test stack flex (Autodesk Fusion 360 design; units mm, degrees)
Autodesk Fusion 360 part; units mm, degrees
sketch "Sketch2" plane through (0, 0, 0) normal (0, 0, 1) x (1, 0, 0) in component "xy"
  line L0 (-95, 0) -> (-95, -95)
  line L1 (-95, -95) -> (0, -95)
  line L2 (0, -20) -> (0, 0)
  line L3 (-38, -95) -> (-38, -47)
  line L4 (-78, -95) -> (-78, -47)
  line L5 (0, 0) -> (-20, 0)
  line L6 (-20, 0) -> (-20, -20)
  line L7 (-20, -20) -> (0, -20)
  line L8 (0, -20) -> (0, 0)
  line L9 (-20, -20) -> (-68, -20)
  line L10 (-110, 0) -> (-110, -110)
  line L11 (-110, -110) -> (0, -110)
  line L12 (-68, -24) -> (-38, -43)
  line L13 (-38, -43) -> (-38, -47)
  line L14 (-38, -47) -> (-78, -47)
  line L15 (0, -95) -> (0, -110)
  line L16 (-95, 0) -> (-110, 0)
  line L17 (-95, 0) -> (-110, 0) construction
  line L18 (0, -110) -> (0, -95) construction
  line L19 (0, -20) -> (0, 0) construction
  line L20 (0, 0) -> (-110, 0) construction
  line L21 (-110, 0) -> (-110, -110) construction
  line L22 (-110, -110) -> (0, -110) construction
  line L23 (0, -110) -> (0, 0) construction
  line L24 (-58, -47) -> (-58, -95) construction
  line L25 (-58.625, -71) -> (-57.375, -71) construction
  line L26 (-58.625, -47) -> (-58.625, -95)
  line L27 (-57.375, -95) -> (-57.375, -47)
  line L28 (-39.25, -95) -> (-39.25, -47)
  line L29 (-76.75, -95) -> (-76.75, -47)
  line L30 (-20, -18.75) -> (-68, -18.75)
  line L31 (0, 0) -> (-20, 0)
  line L32 (-190, 0) -> (-210, 0) construction
  line L33 (-20, 0.625) -> (-68, 0.625)
  line L34 (-20, -0.625) -> (-68, -0.625)
  line L35 (-44, -0.625) -> (-44, 0.625) construction
  line L36 (-20, 0.625) -> (-20, 0)
  line L37 (-20, 18.75) -> (-68, 18.75)
  line L38 (-20, 20) -> (-68, 20)
  line L39 (-78, -47) -> (-78, 20)
  line L40 (-78, 20) -> (-68, 20)
  line L41 (-68, 20) -> (-68, -24)
  line L42 (-20, 18.75) -> (-20, 20)
  line L43 (-20, 20) -> (-20, -18.75)
  line L44 (-20, -20) -> (20, -20)
  line L45 (20, -20) -> (20, 20)
  line L46 (20, 20) -> (-20, 20)
  line L47 (-20, 20) -> (-20, -20)
  line L48 (-20, -20) -> (20, 20) construction
  line L49 (20, -20) -> (-20, 20) construction
  point P0 (-44, 0)
  dimension "d47" = 40
  dimension "d48" = 17
  dimension "d52" = 15
  dimension "d56" = 4
  dimension "d57" = 110
  dimension "d60" = -1.25
  dimension "d64" = 40
  dimension "d86" = 10
  dimension "d117" = 4
  constraint vertical L0
  constraint horizontal L1
  constraint vertical L2
  constraint coincident L2.end L5.start
  constraint coincident L1 L3.start
  constraint perpendicular L1 L3
  constraint coincident L1 L4.start
  constraint perpendicular L1 L4
  constraint equal L3 L4
  constraint horizontal L5
  constraint vertical L6
  constraint horizontal L7
  constraint vertical L8
  constraint equal L6 L7
  constraint perpendicular L6 L9
  constraint equal L4 L9
  constraint horizontal L31
  constraint vertical L10
  constraint horizontal L11
  constraint vertical L18
  constraint equal L10 L11
  constraint vertical L13
  constraint horizontal L14
  constraint coincident L4.end L14.end
  constraint coincident L3.end L13.end
  constraint collinear L17 L31
  constraint collinear L18 L19
  constraint horizontal L20
  constraint vertical L21
  constraint horizontal L22
  constraint vertical L23
  constraint equal L0 L1
  constraint midpoint L14 L24.start
  constraint coincident L1 L24.end
  constraint perpendicular L1 L24
  constraint perpendicular L24 L25
  constraint midpoint L24 L25
  constraint coincident L14 L26.start
  constraint coincident L1 L26.end
  constraint perpendicular L1 L26
  constraint coincident L1 L27.start
  constraint coincident L14 L27.end
  constraint perpendicular L14 L27
  constraint coincident L25.start L26
  constraint coincident L25.end L27
  constraint horizontal L33
  constraint parallel L33 L34
  constraint midpoint L34 L35.start
  constraint coincident L33 L35.end
  constraint perpendicular L33 L35
  constraint midpoint L33 L35.end
  constraint equal L33 L34
  constraint coincident L6 L34.start
  constraint midpoint L35 P0
  constraint coincident L20 P0
  constraint symmetric L6.end L20 L38.start
  constraint symmetric L9.end L20 L38.end
  constraint symmetric L20 L30.start L37.start
  constraint symmetric L20 L30.end L37.end
  constraint vertical L39
  constraint horizontal L40
  constraint vertical L41
  constraint coincident L38.end L40.end
  constraint perpendicular L38 L42
  constraint horizontal L44
  constraint perpendicular L44 L45
  constraint parallel L44 L46
  constraint parallel L45 L47
  constraint coincident L48 L2.end
  constraint coincident L49 L2.end
  constraint coincident L33.end L41
  measures "d47" distance of L3 L4
  measures "d48" distance of L0.end L4
  measures "d52" distance of L0 L10
  measures "d56" distance of L9.end L12.start
  measures "d57" distance of L10.start L10.end
  measures "d86" distance of L12.start L39
  measures "d117" distance of L12.end L3.end
extrude "Extrude3" add sketch "Sketch2" along normal mid plane 80.6636 contours L2 L5 L8 L31 L36 L42 L43 L44 L45 L46 L47 | L2 L5 L6 L7 L8 L31 L43 L44 L47 makes body 1 in component "xy"
extrude "Extrude2" add sketch "Sketch2" along normal mid plane 80.6636 separate body contours L0 L1 L10 L11 L15 L16 | L1 L4 L14 L29 | L12 L13 L14 L39 L40 L41 | L1 L14 L26 L27 | L37 L38 L41 L42 L43 L47 | L1 L3 L14 L28 | L6 L33 L34 L36 L41 L43 L47 | L6 L9 L30 L41 L47 makes body 2 in component "xy"
combine "Combine2" operation add target body 1 tool bodies 2 in component "xy"
fillet "Fillet2" radius 5.558 19 edges at (-20, -18.75, 0) (-20, 0.625, 0) (-20, 18.75, 0) (-20, -0.625, 0) (-68, -18.75, 0) (-68, -20, 0) (-68, 0.625, 0) (-68, -0.625, 0) (-68, 18.75, 0) (-38, -95, 0) (-57.375, -95, 0) (-76.75, -95, 0) (-78, -95, 0) (-39.25, -95, 0) (-58.625, -95, 0) (-76.75, -47, 0) (-57.375, -47, 0) (-39.25, -47, 0) (-58.625, -47, 0) on bodies 1 in component "xy"
pattern_circular "C-Pattern3" count 4 over 360 about axis through (0, 0, 1.75) along (0, 0, 1) of bodies 1 makes body 3 at (110, -36.6667, 13.4439) makes body 4 at (36.6667, 110, 13.4439) makes body 5 at (-110, 36.6667, 13.4439) in component "xy"
combine "Combine3" operation add target body 3 tool bodies 1 5 4 in component "xy"
fillet "Fillet4" radius 6.013 4 edges at (-20, 20, 0) (20, 20, 0) (20, -20, 0) (-20, -20, 0) on bodies 3 in component "xy"
sketch "Sketch3" plane through (0, 0, 40.3318) normal (0, 0, 1) x (-1, 0, 0) in component "xy"
  line L0 (-110, -110) -> (110, -110)
  line L1 (110, -110) -> (110, 110)
  line L2 (110, 110) -> (-110, 110)
  line L3 (-110, 110) -> (-110, -110)
  line L4 (-95, -95) -> (-95, 32.442)
  arc A0 (-89.442, 38) -> (-95, 32.442) centre (-89.442, 32.442) ccw
  line L5 (-89.442, 38) -> (-43, 38)
  line L6 (-43, 38) -> (-24, 68)
  arc A1 (-20, 62.6648) -> (-24, 68) centre (-25.558, 62.6648) ccw
  line L7 (-20, 62.6648) -> (-20, 26.013)
  arc A2 (-26.013, 20) -> (-20, 26.013) centre (-26.013, 26.013) ccw
  line L8 (-26.013, 20) -> (-78, 20)
  line L9 (-78, 20) -> (-78, -89.442)
  arc A3 (-83.558, -95) -> (-78, -89.442) centre (-83.558, -89.442) ccw
  line L10 (-83.558, -95) -> (-95, -95)
  line L11 (-20, 13.192) -> (-20, 6.183)
  arc A4 (-25.558, 0.625) -> (-20, 6.183) centre (-25.558, 6.183) ccw
  line L12 (-25.558, 0.625) -> (-62.442, 0.625)
  arc A5 (-68, 6.183) -> (-62.442, 0.625) centre (-62.442, 6.183) ccw
  line L13 (-68, 6.183) -> (-68, 13.192)
  arc A6 (-62.442, 18.75) -> (-68, 13.192) centre (-62.442, 13.192) ccw
  line L14 (-62.442, 18.75) -> (-25.558, 18.75)
  arc A7 (-20, 13.192) -> (-25.558, 18.75) centre (-25.558, 13.192) ccw
  line L15 (-20, -6.183) -> (-20, -13.192)
  arc A8 (-25.558, -18.75) -> (-20, -13.192) centre (-25.558, -13.192) ccw
  line L16 (-25.558, -18.75) -> (-62.442, -18.75)
  arc A9 (-68, -13.192) -> (-62.442, -18.75) centre (-62.442, -13.192) ccw
  line L17 (-68, -13.192) -> (-68, -6.183)
  arc A10 (-62.442, -0.625) -> (-68, -6.183) centre (-62.442, -6.183) ccw
  line L18 (-62.442, -0.625) -> (-25.558, -0.625)
  arc A11 (-20, -6.183) -> (-25.558, -0.625) centre (-25.558, -6.183) ccw
  line L19 (-44.808, -95) -> (-51.817, -95)
  arc A12 (-57.375, -89.442) -> (-51.817, -95) centre (-51.817, -89.442) ccw
  line L20 (-57.375, -89.442) -> (-57.375, -52.558)
  arc A13 (-51.817, -47) -> (-57.375, -52.558) centre (-51.817, -52.558) ccw
  line L21 (-51.817, -47) -> (-44.808, -47)
  arc A14 (-39.25, -52.558) -> (-44.808, -47) centre (-44.808, -52.558) ccw
  line L22 (-39.25, -52.558) -> (-39.25, -89.442)
  arc A15 (-44.808, -95) -> (-39.25, -89.442) centre (-44.808, -89.442) ccw
  line L23 (-71.192, -47) -> (-64.183, -47)
  arc A16 (-58.625, -52.558) -> (-64.183, -47) centre (-64.183, -52.558) ccw
  line L24 (-58.625, -52.558) -> (-58.625, -89.442)
  arc A17 (-64.183, -95) -> (-58.625, -89.442) centre (-64.183, -89.442) ccw
  line L25 (-64.183, -95) -> (-71.192, -95)
  arc A18 (-76.75, -89.442) -> (-71.192, -95) centre (-71.192, -89.442) ccw
  line L26 (-76.75, -89.442) -> (-76.75, -52.558)
  arc A19 (-71.192, -47) -> (-76.75, -52.558) centre (-71.192, -52.558) ccw
  arc A20 (-18.75, 25.558) -> (-13.192, 20) centre (-13.192, 25.558) ccw
  line L27 (-18.75, 25.558) -> (-18.75, 62.442)
  arc A21 (-13.192, 68) -> (-18.75, 62.442) centre (-13.192, 62.442) ccw
  line L28 (-13.192, 68) -> (-6.183, 68)
  arc A22 (-0.625, 62.442) -> (-6.183, 68) centre (-6.183, 62.442) ccw
  line L29 (-0.625, 62.442) -> (-0.625, 25.558)
  arc A23 (-6.183, 20) -> (-0.625, 25.558) centre (-6.183, 25.558) ccw
  line L30 (-6.183, 20) -> (-13.192, 20)
  arc A24 (0.625, 25.558) -> (6.183, 20) centre (6.183, 25.558) ccw
  line L31 (0.625, 25.558) -> (0.625, 62.442)
  arc A25 (6.183, 68) -> (0.625, 62.442) centre (6.183, 62.442) ccw
  line L32 (6.183, 68) -> (13.192, 68)
  arc A26 (18.75, 62.442) -> (13.192, 68) centre (13.192, 62.442) ccw
  line L33 (18.75, 62.442) -> (18.75, 25.558)
  arc A27 (13.192, 20) -> (18.75, 25.558) centre (13.192, 25.558) ccw
  line L34 (13.192, 20) -> (6.183, 20)
  line L35 (20, 26.013) -> (20, 78)
  line L36 (20, 78) -> (-89.442, 78)
  arc A28 (-95, 83.558) -> (-89.442, 78) centre (-89.442, 83.558) ccw
  line L37 (-95, 83.558) -> (-95, 95)
  line L38 (-95, 95) -> (32.442, 95)
  arc A29 (38, 89.442) -> (32.442, 95) centre (32.442, 89.442) ccw
  line L39 (38, 89.442) -> (38, 43)
  line L40 (38, 43) -> (68, 24)
  arc A30 (62.6648, 20) -> (68, 24) centre (62.6648, 25.558) ccw
  line L41 (62.6648, 20) -> (26.013, 20)
  arc A31 (20, 26.013) -> (26.013, 20) centre (26.013, 26.013) ccw
  line L42 (95, -95) -> (-32.442, -95)
  arc A32 (-38, -89.442) -> (-32.442, -95) centre (-32.442, -89.442) ccw
  line L43 (-38, -89.442) -> (-38, -43)
  line L44 (-38, -43) -> (-68, -24)
  arc A33 (-62.6648, -20) -> (-68, -24) centre (-62.6648, -25.558) ccw
  line L45 (-62.6648, -20) -> (-26.013, -20)
  arc A34 (-20, -26.013) -> (-26.013, -20) centre (-26.013, -26.013) ccw
  line L46 (-20, -26.013) -> (-20, -78)
  line L47 (-20, -78) -> (89.442, -78)
  arc A35 (95, -83.558) -> (89.442, -78) centre (89.442, -83.558) ccw
  line L48 (95, -83.558) -> (95, -95)
  arc A36 (25.558, 18.75) -> (20, 13.192) centre (25.558, 13.192) ccw
  line L49 (25.558, 18.75) -> (62.442, 18.75)
  arc A37 (68, 13.192) -> (62.442, 18.75) centre (62.442, 13.192) ccw
  line L50 (68, 13.192) -> (68, 6.183)
  arc A38 (62.442, 0.625) -> (68, 6.183) centre (62.442, 6.183) ccw
  line L51 (62.442, 0.625) -> (25.558, 0.625)
  arc A39 (20, 6.183) -> (25.558, 0.625) centre (25.558, 6.183) ccw
  line L52 (20, 6.183) -> (20, 13.192)
  line L53 (-13.192, -20) -> (-6.183, -20)
  arc A40 (-0.625, -25.558) -> (-6.183, -20) centre (-6.183, -25.558) ccw
  line L54 (-0.625, -25.558) -> (-0.625, -62.442)
  arc A41 (-6.183, -68) -> (-0.625, -62.442) centre (-6.183, -62.442) ccw
  line L55 (-6.183, -68) -> (-13.192, -68)
  arc A42 (-18.75, -62.442) -> (-13.192, -68) centre (-13.192, -62.442) ccw
  line L56 (-18.75, -62.442) -> (-18.75, -25.558)
  arc A43 (-13.192, -20) -> (-18.75, -25.558) centre (-13.192, -25.558) ccw
  arc A44 (25.558, -0.625) -> (20, -6.183) centre (25.558, -6.183) ccw
  line L57 (25.558, -0.625) -> (62.442, -0.625)
  arc A45 (68, -6.183) -> (62.442, -0.625) centre (62.442, -6.183) ccw
  line L58 (68, -6.183) -> (68, -13.192)
  arc A46 (62.442, -18.75) -> (68, -13.192) centre (62.442, -13.192) ccw
  line L59 (62.442, -18.75) -> (25.558, -18.75)
  arc A47 (20, -13.192) -> (25.558, -18.75) centre (25.558, -13.192) ccw
  line L60 (20, -13.192) -> (20, -6.183)
  line L61 (6.183, -20) -> (13.192, -20)
  arc A48 (18.75, -25.558) -> (13.192, -20) centre (13.192, -25.558) ccw
  line L62 (18.75, -25.558) -> (18.75, -62.442)
  arc A49 (13.192, -68) -> (18.75, -62.442) centre (13.192, -62.442) ccw
  line L63 (13.192, -68) -> (6.183, -68)
  arc A50 (0.625, -62.442) -> (6.183, -68) centre (6.183, -62.442) ccw
  line L64 (0.625, -62.442) -> (0.625, -25.558)
  arc A51 (6.183, -20) -> (0.625, -25.558) centre (6.183, -25.558) ccw
  line L65 (-95, 44.808) -> (-95, 51.817)
  arc A52 (-89.442, 57.375) -> (-95, 51.817) centre (-89.442, 51.817) ccw
  line L66 (-89.442, 57.375) -> (-52.558, 57.375)
  arc A53 (-47, 51.817) -> (-52.558, 57.375) centre (-52.558, 51.817) ccw
  line L67 (-47, 51.817) -> (-47, 44.808)
  arc A54 (-52.558, 39.25) -> (-47, 44.808) centre (-52.558, 44.808) ccw
  line L68 (-52.558, 39.25) -> (-89.442, 39.25)
  arc A55 (-95, 44.808) -> (-89.442, 39.25) centre (-89.442, 44.808) ccw
  line L69 (-47, 71.192) -> (-47, 64.183)
  arc A56 (-52.558, 58.625) -> (-47, 64.183) centre (-52.558, 64.183) ccw
  line L70 (-52.558, 58.625) -> (-89.442, 58.625)
  arc A57 (-95, 64.183) -> (-89.442, 58.625) centre (-89.442, 64.183) ccw
  line L71 (-95, 64.183) -> (-95, 71.192)
  arc A58 (-89.442, 76.75) -> (-95, 71.192) centre (-89.442, 71.192) ccw
  line L72 (-89.442, 76.75) -> (-52.558, 76.75)
  arc A59 (-47, 71.192) -> (-52.558, 76.75) centre (-52.558, 71.192) ccw
  line L73 (44.808, 95) -> (51.817, 95)
  arc A60 (57.375, 89.442) -> (51.817, 95) centre (51.817, 89.442) ccw
  line L74 (57.375, 89.442) -> (57.375, 52.558)
  arc A61 (51.817, 47) -> (57.375, 52.558) centre (51.817, 52.558) ccw
  line L75 (51.817, 47) -> (44.808, 47)
  arc A62 (39.25, 52.558) -> (44.808, 47) centre (44.808, 52.558) ccw
  line L76 (39.25, 52.558) -> (39.25, 89.442)
  arc A63 (44.808, 95) -> (39.25, 89.442) centre (44.808, 89.442) ccw
  line L77 (71.192, 47) -> (64.183, 47)
  arc A64 (58.625, 52.558) -> (64.183, 47) centre (64.183, 52.558) ccw
  line L78 (58.625, 52.558) -> (58.625, 89.442)
  arc A65 (64.183, 95) -> (58.625, 89.442) centre (64.183, 89.442) ccw
  line L79 (64.183, 95) -> (71.192, 95)
  arc A66 (76.75, 89.442) -> (71.192, 95) centre (71.192, 89.442) ccw
  line L80 (76.75, 89.442) -> (76.75, 52.558)
  arc A67 (71.192, 47) -> (76.75, 52.558) centre (71.192, 52.558) ccw
  line L81 (47, -71.192) -> (47, -64.183)
  arc A68 (52.558, -58.625) -> (47, -64.183) centre (52.558, -64.183) ccw
  line L82 (52.558, -58.625) -> (89.442, -58.625)
  arc A69 (95, -64.183) -> (89.442, -58.625) centre (89.442, -64.183) ccw
  line L83 (95, -64.183) -> (95, -71.192)
  arc A70 (89.442, -76.75) -> (95, -71.192) centre (89.442, -71.192) ccw
  line L84 (89.442, -76.75) -> (52.558, -76.75)
  arc A71 (47, -71.192) -> (52.558, -76.75) centre (52.558, -71.192) ccw
  line L85 (95, -44.808) -> (95, -51.817)
  arc A72 (89.442, -57.375) -> (95, -51.817) centre (89.442, -51.817) ccw
  line L86 (89.442, -57.375) -> (52.558, -57.375)
  arc A73 (47, -51.817) -> (52.558, -57.375) centre (52.558, -51.817) ccw
  line L87 (47, -51.817) -> (47, -44.808)
  arc A74 (52.558, -39.25) -> (47, -44.808) centre (52.558, -44.808) ccw
  line L88 (52.558, -39.25) -> (89.442, -39.25)
  arc A75 (95, -44.808) -> (89.442, -39.25) centre (89.442, -44.808) ccw
  line L89 (26.013, -20) -> (78, -20)
  line L90 (78, -20) -> (78, 89.442)
  arc A76 (83.558, 95) -> (78, 89.442) centre (83.558, 89.442) ccw
  line L91 (83.558, 95) -> (95, 95)
  line L92 (95, 95) -> (95, -32.442)
  arc A77 (89.442, -38) -> (95, -32.442) centre (89.442, -32.442) ccw
  line L93 (89.442, -38) -> (43, -38)
  line L94 (43, -38) -> (24, -68)
  arc A78 (20, -62.6648) -> (24, -68) centre (25.558, -62.6648) ccw
  line L95 (20, -62.6648) -> (20, -26.013)
  arc A79 (26.013, -20) -> (20, -26.013) centre (26.013, -26.013) ccw
  line L96 (-20, 20) -> (20, 20)
  line L97 (20, 20) -> (20, -20)
  line L98 (20, -20) -> (-20, -20)
  line L99 (-20, -20) -> (-20, 20)
  line L100 (-20, 20) -> (20, -20) construction
  line L101 (20, 20) -> (-20, -20) construction
  line L102 (-95, 95) -> (95, 95)
  line L103 (95, 95) -> (95, -95)
  line L104 (95, -95) -> (-95, -95)
  line L105 (-95, -95) -> (-95, 95)
  line L106 (-95, 95) -> (95, -95) construction
  line L107 (95, 95) -> (-95, -95) construction
  line L108 (-110, 110) -> (110, 110)
  line L109 (110, 110) -> (110, -110)
  line L110 (110, -110) -> (-110, -110)
  line L111 (-110, -110) -> (-110, 110)
  line L112 (-110, 110) -> (110, -110) construction
  line L113 (110, 110) -> (-110, -110) construction
  constraint horizontal L96
  constraint perpendicular L96 L97
  constraint parallel L96 L98
  constraint parallel L97 L99
  constraint coincident L100 origin
  constraint coincident L101 origin
  constraint horizontal L102
  constraint perpendicular L102 L103
  constraint parallel L102 L104
  constraint parallel L103 L105
  constraint coincident L106 origin
  constraint coincident L107 origin
  constraint coincident L37.end L38.start
  constraint horizontal L108
  constraint perpendicular L108 L109
  constraint parallel L108 L110
  constraint parallel L109 L111
  constraint coincident L112 origin
  constraint coincident L113 origin
  constraint coincident L2.end L3.start
extrude "Extrude4" add sketch "Sketch3" along normal blind 1 contours L0 L1 L2 L3 L108 L109 L110 L111 | L11 L15 L30 L34 L52 L53 L60 L61 L96 L97 L98 L99 bodies 3 in component "xy"
sketch "Sketch2 (1)" plane through (0, 0, 0) normal (0, 0, 1) x (1, 0, 0) in component "xy"
pattern_linear "R-Pattern1" count 3 spacing 101.8223 along (0, 0, 1) of bodies 3 makes body 6 at (-1.539, -6.7417, 61.4905) makes body 7 at (-1.539, -6.7417, 163.3128) in component "xy"
extrude "Extrude5" add 1 faces at (6.6667, -6.6667, 41.3318) along direction (0, 0, 1) blind 57.85 on bodies 3 bodies 3 6 in component "xy"
extrude "Extrude6" add 1 faces at (105, -31.6667, 143.1541) along direction (0, 0, 1) blind 28.192 on bodies 3 bodies 3 7 in component "xy"
component "Configuration 1 v12" placed x (1, 0, 0) y (0, 1, 0) z (0, 0, 1) at (0, 0, 0)
component "xy" placed x (1, 0, 0) y (0, 1, 0) z (0, 0, 1) at (0, 0, 0) in component "Configuration 1 v12"
equation "travle_xy = 15 mm"
equation "ofset_xy_travle = 2 mm"
equation "stage_size = 40 mm"
equation "zy_suqare_box = 220 mm"
equation "zy_flex_thicknes = -1.25 mm"
equation "xy_flex_down_extrude = 50 mm"
equation "stage_xy_intermideaat_body = 10 mm"
equation "d47 = stage_size"
equation "d48 = ofset_xy_travle + travle_xy"
equation "d56 = d64 / 10"
equation "d57 = zy_suqare_box / 2"
equation "d59 = -zy_flex_thicknes"
equation "d60 = zy_flex_thicknes"
equation "d61 = -zy_flex_thicknes"
equation "d62 = -zy_flex_thicknes"
equation "d64 = stage_size"
equation "d69 = -zy_flex_thicknes"
equation "d70 = d76"
equation "zy_flex_filet = 15 mm"
equation "d76 = 80.6635685442 mm"
equation "d86 = stage_xy_intermideaat_body"
equation "scrue_top_stage = 130 mm"
equation "scrue_langth = 200 mm"
equation "roatate_flex_thick = 1 mm"
equation "decoupling_filit_radies = 3.0026285896 mm"
equation "d117 = d56"
